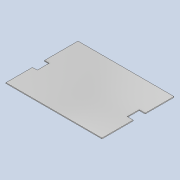
# Autodesk Inventor part: Stock Aluminum Sheet
Saved by Autodesk Inventor 2022 (Build 260153000, 153)
## iProperties
Created: 2021-10-30
Part Number: Stock Aluminum Sheet
Material: Generic
Document SubType Name: Modeling
Designer: Coy
Density: 1 g/cm^3
Appearance: Machined - Aluminum
Author: Coy
Autodesk Inventor part; units mm, degrees
ref_plane "YZ Plane" through (0, 0, 0) normal (1, 0, 0) x (0, 1, 0)
ref_plane "XZ Plane" through (0, 0, 0) normal (0, 1, 0) x (-1, 0, 0)
ref_plane "XY Plane" through (0, 0, 0) normal (0, 0, 1) x (1, 0, 0)
sketch "Sketch1" plane through (0, 0, 0) normal (0, 1, 0) x (-1, 0, 0)
  line L0 (0, 0) -> (400, 0)
  line L1 (400, 0) -> (400, 300)
  line L2 (400, 300) -> (0, 300)
  line L3 (0, 300) -> (0, 0)
  dimension "d0" = 300
  dimension "d1" = 400
  constraints: 8 end point, 2 parallel, 1 horizontal, 1 perpendicular
  measures "d0" distance of L2.end L0.start
  measures "d1" distance of L0.start L0.end
extrude "Extrusion1" add sketch "Sketch1" along normal blind 3.175
sketch "Sketch2" plane through (0, 3.175, 0) normal (0, 1, 0) x (1, 0, 0)
  line L0 (0, -300) -> (0, 0) projected
  line L1 (0, -170) -> (-25, -170)
  line L2 (-25, -170) -> (-25, -120)
  line L3 (-25, -120) -> (0, -120)
  line L4 (0, -120) -> (0, -170)
  line L5 (-400, 0) -> (-400, -300) projected
  line L6 (-400, -190) -> (-380, -190)
  line L7 (-380, -190) -> (-380, -140)
  line L8 (-380, -140) -> (-400, -140)
  line L9 (-400, -140) -> (-400, -190)
  line L10 (-400, -300) -> (0, -300) projected
  point P0 (0, -120)
  dimension "d4" = 25
  dimension "d5" = 130
  dimension "d6" = 180
  dimension "d7" = 20
  dimension "d8" = 110
  dimension "d9" = 160
  constraints: 16 end point, 4 parallel, 2 horizontal, 2 perpendicular, 2 point on line
  measures "d4" distance of L1.start L1.end
  measures "d5" distance between parallel lines of L10 L1
  measures "d6" distance between parallel lines of L10 L3
  measures "d7" distance of L6.start L6.end
  measures "d8" distance between parallel lines of L10 L6
  measures "d9" distance from line of L5.end L8
extrude "Extrusion2" cut sketch "Sketch2" against normal through all
body "Solid1"
